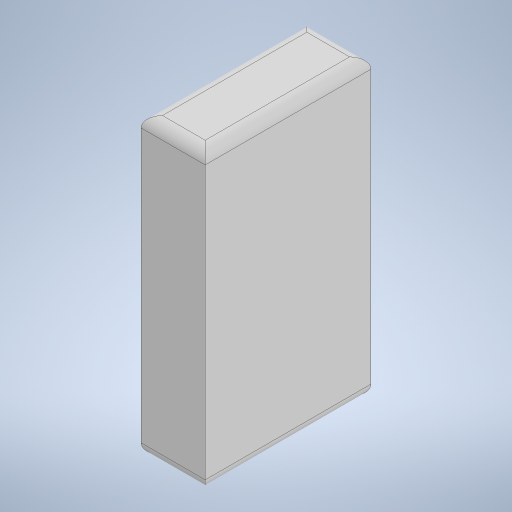
# Autodesk Inventor part: Battery
Saved by Autodesk Inventor 2024 (Build 280153000, 153)
## iProperties
Created: 2024-04-25
Part Number: Battery
Material: Generic
Document SubType Name: Modeling
Designer: auror
Density: 1 g/cm^3
Appearance: Default
Author: auror
Autodesk Inventor part; units mm, degrees
ref_plane "YZ Plane" through (0, 0, 0) normal (1, 0, 0) x (0, 1, 0)
ref_plane "XZ Plane" through (0, 0, 0) normal (0, 1, 0) x (-1, 0, 0)
ref_plane "XY Plane" through (0, 0, 0) normal (0, 0, 1) x (1, 0, 0)
sketch "Sketch1" plane through (0, 0, 0) normal (0, 1, 0) x (-1, 0, 0)
  line L0 (8.2178, 17.3206) -> (-3.7822, 17.3206)
  line L1 (-3.7822, 17.3206) -> (-3.7822, -13.6794)
  line L2 (-3.7822, -13.6794) -> (8.2178, -13.6794)
  line L3 (8.2178, -13.6794) -> (8.2178, 17.3206)
  point P0 (0, 0)
  dimension "d0" = 31
  dimension "d1" = 12
  constraints: 8 end point, 2 parallel, 1 horizontal, 1 perpendicular
  measures "d0" distance of L2.end L0.start
  measures "d1" distance of L0.start L0.end
extrude "Extrusion1" add sketch "Sketch1" along normal blind 55
fillet "Fillet1" radius 2 8 edges at (-2.2178, 55, 17.3206) (3.7822, 55, 1.8206) (-2.2178, 55, -13.6794) (-8.2178, 55, 1.8206) (3.7822, 0, 1.8206) (-2.2178, 0, 17.3206) (-2.2178, 0, -13.6794) (-8.2178, 0, 1.8206)
body "Solid1"
